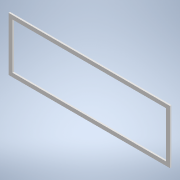
# Autodesk Inventor part: PrimaryCoilAluminiumLayer
Saved by Autodesk Inventor 2021 (Build 250183000, 183)
## iProperties
Created: 2022-01-19
Part Number: PrimaryCoilAluminiumLayer
Material: Silver
Document SubType Name: Modeling
Designer: avan411
Density: 10.49 g/cm^3
Appearance: Silver
Author: avan411
Autodesk Inventor part; units mm, degrees
ref_plane "YZ Plane" through (0, 0, 0) normal (1, 0, 0) x (0, 1, 0)
ref_plane "XZ Plane" through (0, 0, 0) normal (0, 1, 0) x (-1, 0, 0)
ref_plane "XY Plane" through (0, 0, 0) normal (0, 0, 1) x (1, 0, 0)
sketch "Sketch1" plane through (0, 0, 0) normal (0, 0, 1) x (1, 0, 0)
  line L0 (97.5839, -20.2585) -> (97.5839, -84.5585) construction
  line L1 (97.5839, -52.4085) -> (19.6066, -52.4085)
  line L2 (622.5839, -227.4085) -> (-427.4161, -227.4085)
  line L3 (-427.4161, -227.4085) -> (-427.4161, 122.5915)
  line L4 (-427.4161, 122.5915) -> (622.5839, 122.5915)
  line L5 (622.5839, 122.5915) -> (622.5839, -227.4085)
  line L6 (622.5839, -227.4085) -> (-427.4161, 122.5915) construction
  line L7 (-427.4161, -227.4085) -> (622.5839, 122.5915) construction
  line L8 (-402.4161, 97.5915) -> (597.5839, 97.5915)
  line L9 (597.5839, 97.5915) -> (597.5839, -202.4085)
  line L10 (597.5839, -202.4085) -> (-402.4161, -202.4085)
  line L11 (-402.4161, -202.4085) -> (-402.4161, 97.5915)
  line L12 (-402.4161, 97.5915) -> (597.5839, -202.4085) construction
  line L13 (597.5839, 97.5915) -> (-402.4161, -202.4085) construction
  circle A0 centre (-417.4161, -217.4085) radius 3 projected
  circle A1 centre (-159.9161, -217.4085) radius 3 projected
  circle A2 centre (97.5839, 112.5915) radius 3 projected
  circle A3 centre (-159.9161, 112.5915) radius 3 projected
  circle A4 centre (-417.4161, 112.5915) radius 3 projected
  circle A5 centre (355.0839, 112.5915) radius 3 projected
  circle A6 centre (612.5839, 112.5915) radius 3 projected
  circle A7 centre (612.5839, -217.4085) radius 3 projected
  circle A8 centre (355.0839, -217.4085) radius 3 projected
  circle A9 centre (97.5839, -217.4085) radius 3 projected
  point P0 (0, 0)
  dimension "d0" = 1050
  dimension "d1" = 350
  dimension "d6" = 1000
  dimension "d7" = 300
  constraints: 28 end point, 5 midpoint, 4 parallel, 2 horizontal, 2 perpendicular
  measures "d0" distance of L3.end L4.end
  measures "d1" distance of L2.end L3.end
  measures "d6" distance of L9.end L10.end
  measures "d7" distance of L10.end L8.start
extrude "Extrusion2" add sketch "Sketch1" along normal blind 4
body "Solid2"
